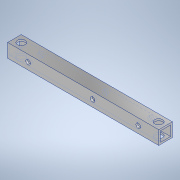
# Autodesk Inventor part: ロボット回転9ｘ9_1
Saved by Autodesk Inventor 2020.3 (Build 243373000, 373)
## iProperties
Created: 2020-07-04
Part Number: ロボット回転9ｘ9_1
Material: アルミニウム 6061
Document SubType Name: Modeling
Designer: totot
Density: 2.7 g/cm^3
Appearance: アルミニウム - フラット
Mass: 9.71316 g
Surface Area: 61.9129 cm^2
Volume: 3.59746 cm^3
Author: totot
Autodesk Inventor part; units mm, degrees
ref_plane "YZ Plane" through (0, 0, 0) normal (1, 0, 0) x (0, 1, 0)
ref_plane "XZ Plane" through (0, 0, 0) normal (0, 1, 0) x (-1, 0, 0)
ref_plane "XY Plane" through (0, 0, 0) normal (0, 0, 1) x (1, 0, 0)
sketch "スケッチ1" plane through (0, 0, 0) normal (1, 0, 0) x (0, 1, 0)
  line L0 (0, 0) -> (9, 0)
  line L1 (9, 0) -> (9, -9)
  line L2 (9, -9) -> (0, -9)
  line L3 (0, -9) -> (0, 0)
  line L4 (1.2, -1.2) -> (7.8, -1.2)
  line L5 (7.8, -1.2) -> (7.8, -7.8)
  line L6 (7.8, -7.8) -> (1.2, -7.8)
  line L7 (1.2, -7.8) -> (1.2, -1.2)
  dimension "d0" = 9
  dimension "d1" = 9
  dimension "d2" = 1.2
  dimension "d3" = 1.2
  dimension "d4" = 1.2
  dimension "d5" = 1.2
  constraints: 16 end point, 4 parallel, 2 horizontal, 2 perpendicular
  measures "d0" distance of L1.end L2.end
  measures "d1" distance of L0.end L1.end
  measures "d2" distance between parallel lines of L2 L6
  measures "d3" distance between parallel lines of L0 L4
  measures "d4" distance between parallel lines of L7 L3
  measures "d5" distance between parallel lines of L1 L5
extrude "押し出し1" add sketch "スケッチ1" along normal blind 99.5097
sketch "スケッチ2" plane through (0, 0, -9) normal (0, -1, 0) x (1, 0, 0)
  line L0 (0, 9) -> (0, 0) projected
  line L1 (99.5097, 9) -> (99.5097, 0) projected
  line L2 (0, 9) -> (99.5097, 9) projected
  point P0 (95.0097, 4.5)
  point P1 (4.5, 4.5)
  dimension "d8" = 4.5
  dimension "d9" = 4.5
  dimension "d10" = 4.5
  dimension "d11" = 4.5
  measures "d8" distance from line of point (4.5, 4.5) L0
  measures "d9" distance from line of L1 point (95.01, 4.5)
  measures "d10" distance from line of point (4.5, 4.5) L2
  measures "d11" distance from line of L2 point (95.01, 4.5)
hole "穴1" at (95.0097, 0, -4.5) at (4.5, 0, -4.5) direction (0, 1, 0) diameter 5 end through all
sketch "スケッチ3" plane through (0, 0, 0) normal (0, 0, 1) x (1, 0, 0)
  line L0 (0, 9) -> (0, 0) projected
  line L1 (0, 9) -> (99.5097, 9) projected
  line L2 (99.5097, 9) -> (99.5097, 0) projected
  point P0 (13.5, 4.5)
  point P1 (86.0097, 4.5)
  dimension "d19" = 13.5
  dimension "d20" = 4.5
  dimension "d21" = 4.5
  dimension "d22" = 13.5
  measures "d19" distance from line of point (13.5, 4.5) L0
  measures "d20" distance from line of point (13.5, 4.5) L1
  measures "d21" distance from line of point (86.01, 4.5) L1
  measures "d22" distance from line of point (86.01, 4.5) L2
hole "穴2" at (13.5, 4.5, 0) at (86.0097, 4.5, 0) direction (0, 0, -1) diameter 3 end through all
sketch "スケッチ4" plane through (0, 0, -9) normal (0, 0, -1) x (-1, 0, 0)
  line L0 (0, 0) -> (-99.5097, 0) projected
  circle A0 centre (-86.0097, 4.5) radius 1.5 projected
  point P0 (-56.0097, 4.5)
  dimension "d30" = 4.5
  dimension "d31" = 30
  measures "d30" distance from line of point (-56.01, 4.5) L0
  measures "d31" distance of point (-56.01, 4.5) A0.centre
hole "穴3" at (56.0097, 4.5, -9) direction (0, 0, 1) diameter 3 end through all
equation "\"d3\" = d2"
equation "\"d4\" = d2"
equation "\"d5\" = d4"
equation "\"d9\" = d8"
equation "\"d11\" = d10"
